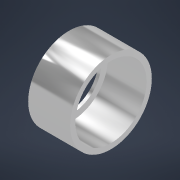
# Autodesk Inventor part: 031
Saved by Autodesk Inventor 2022 (Build 260153000, 153)
## iProperties
Created: 2022-04-04
Part Number: 031
Material: Aluminum 6061
Document SubType Name: Modeling
Designer: Vinicius Miguel
Density: 2.7 g/cm^3
Appearance: Aluminum - Flat
Author: Vinicius Miguel
Autodesk Inventor part; units mm, degrees
ref_plane "YZ Plane" through (0, 0, 0) normal (1, 0, 0) x (0, 1, 0)
ref_plane "XZ Plane" through (0, 0, 0) normal (0, 1, 0) x (-1, 0, 0)
ref_plane "XY Plane" through (0, 0, 0) normal (0, 0, 1) x (1, 0, 0)
sketch "Sketch1" plane through (0, 0, 0) normal (0, 1, 0) x (-1, 0, 0)
  line L0 (0, 0) -> (18, 0)
  line L1 (18, 12.75) -> (18, 19.5)
  line L2 (18, 19.5) -> (0, 19.5)
  line L3 (0, 19.5) -> (0, 17)
  line L4 (0, 17) -> (16.5, 17)
  line L5 (16.5, 17) -> (16.5, 12.75)
  line L6 (16.5, 12.75) -> (18, 12.75)
  dimension "d0" = 34
  dimension "d1" = 2.5
  dimension "d2" = 18
  dimension "d3" = 1.5
  dimension "d6" = 25.5
  constraints: 14 end point, 5 perpendicular, 2 vertical alignment, 1 horizontal, 1 vertical
  measures "d0" diameter of L4 L0
  measures "d1" distance of L2.end L3.end
  measures "d2" distance of L1.end L2.end
  measures "d3" distance of L5.end L1.start
  measures "d6" diameter of L6 L0
revolve "Revolution1" add sketch "Sketch1" angle 360 about axis through (0, 0, 0) along (-1, 0, 0)
chamfer "Chamfer1" distance 1 angle 45 2 edges at (0, 0, -19.5) (-18, 0, -19.5)
body "Solid1"
